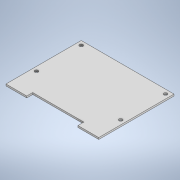
# Autodesk Inventor part: EN715_with_JetsonXavierNX_and_Fan
Saved by Autodesk Inventor 2020.4 (Build 244396000, 396)
## iProperties
Created: 2022-01-24
Part Number: EN715_with_JetsonXavierNX_and_Fan
Material: 一般
Document SubType Name: Modeling
Designer: Masato Kubotera
Density: 1 g/cm^3
Appearance: 既定
Author: Masato Kubotera
Autodesk Inventor part; units mm, degrees
ref_plane "YZ Plane" through (0, 0, 0) normal (1, 0, 0) x (0, 1, 0)
ref_plane "XZ Plane" through (0, 0, 0) normal (0, 1, 0) x (-1, 0, 0)
ref_plane "XY Plane" through (0, 0, 0) normal (0, 0, 1) x (1, 0, 0)
sketch "スケッチ1" plane through (0, 0, 0) normal (0, 0, 1) x (1, 0, 0)
  line L0 (35.3, 43.5) -> (-35.3, 43.5)
  line L1 (-35.3, 43.5) -> (-35.3, -43.5)
  line L2 (-35.3, -43.5) -> (35.3, -43.5)
  line L3 (35.3, -43.5) -> (35.3, 43.5)
  line L4 (35.3, 43.5) -> (-35.3, -43.5) construction
  line L5 (-35.3, 43.5) -> (35.3, -43.5) construction
  line L6 (35.3, 24) -> (29.7, 24)
  line L7 (29.7, 24) -> (29.7, -24)
  line L8 (29.7, -24) -> (35.3, -24)
  line L9 (35.3, 0) -> (-35.3, 0) construction
  line L10 (10.7, -39.5) -> (-31.3, -39.5) construction
  line L11 (-31.3, -39.5) -> (-31.3, 39.5) construction
  line L12 (-31.3, 39.5) -> (10.7, 39.5) construction
  line L13 (10.7, 39.5) -> (10.7, -39.5) construction
  line L14 (10.7, -39.5) -> (-31.3, 39.5) construction
  line L15 (-31.3, -39.5) -> (10.7, 39.5) construction
  circle A0 centre (-31.3, 39.5) radius 1.6
  circle A1 centre (10.7, 39.5) radius 1.6
  circle A2 centre (-31.3, -39.5) radius 1.6
  circle A3 centre (10.7, -39.5) radius 1.6
  point P0 (0, 0)
  point P1 (-10.3, 0)
  dimension "d0" = 70.6
  dimension "d1" = 87
  dimension "d2" = 19.5
  dimension "d3" = 48
  dimension "d4" = 65
  dimension "d5" = 4
  dimension "d6" = 4
  dimension "d7" = 46
  dimension "d8" = 3.2
  dimension "d9" = 3.2
  constraints: 32 end point, 6 midpoint, 4 centre point, 4 parallel, 4 perpendicular, 3 horizontal, 3 point on line, 2 coincident, 2 symmetric about line, 3 other
  measures "d0" distance of L2.end L1.end
  measures "d1" distance of L1.end L0.end
  measures "d2" distance of L0.start L6.start
  measures "d3" distance of L8.end L6.start
  measures "d4" horizontal distance of L0.end L6.end
  measures "d5" horizontal distance of L11.end L0.end
  measures "d6" horizontal distance of L0.end L11.end
  measures "d7" horizontal distance of L0.end L12.end
  measures "d8" diameter of A0
  measures "d9" diameter of A1
extrude "押し出し1" add sketch "スケッチ1" along normal blind 1.6 contours L3 L6 L7 L8 L2 L1 L0
equation "\"d9\" = d8"
